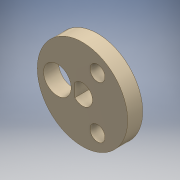
# Autodesk Inventor part: Carrier_top
Saved by Autodesk Inventor 2016 (Build 200138000, 138)
## iProperties
Created: 2015-12-09
Part Number: Carrier_top
Material: Generic
Document SubType Name: Modeling
Designer: lk8187
Density: 1 g/cm^3
Appearance: Smooth - Light Beige
Author: lk8187
Autodesk Inventor part; units mm, degrees
ref_plane "YZ Plane" through (0, 0, 0) normal (1, 0, 0) x (0, 1, 0)
ref_plane "XZ Plane" through (0, 0, 0) normal (0, 1, 0) x (-1, 0, 0)
ref_plane "XY Plane" through (0, 0, 0) normal (0, 0, 1) x (1, 0, 0)
sketch "Sketch1" plane through (0, 0, 0) normal (0, 1, 0) x (-1, 0, 0)
  circle A0 centre (0, 0) radius 9
  circle A1 centre (5, 0) radius 6 construction
  line L0 (0, 0) -> (-3, -5.1962) construction
  line L1 (0, 0) -> (-3, 5.1962) construction
  line L2 (0, 0) -> (-6.6506, 0) construction
  circle A2 centre (-3, 5.1962) radius 1.5
  circle A3 centre (-3, -5.1962) radius 1.5
  circle A4 centre (5, 0) radius 2.75
  arc A5 (1.5, 1.3229) -> (1.5, -1.3229) centre (0, 0) ccw
  line L3 (1.5, 1.3229) -> (1.5, -1.3229)
  dimension "d0" = 18
  dimension "d1" = 5
  dimension "d2" = 12
  dimension "d3" = 60
  dimension "d4" = 6
  dimension "d5" = 3
  dimension "d6" = 3
  dimension "d7" = 5.5
  dimension "d9" = 4
  dimension "d10" = 1.5
  constraints: 8 end point, 6 centre point, 5 coincident, 2 point on circle, 1 equal length, 1 horizontal, 1 horizontal alignment, 1 vertical, 1 vertical alignment
  measures "d0" diameter of A0
  measures "d1" distance of A1.centre point (0, 0)
  measures "d2" diameter of A1
  measures "d3" angle of L2 L0
  measures "d4" distance of L0.start L0.end
  measures "d5" diameter of A3
  measures "d6" diameter of A2
  measures "d7" diameter of A4
  measures "d9" diameter of A5
  measures "d10" distance from line of L3 point (0, 0)
extrude "Extrusion1" add sketch "Sketch1" against normal blind 3
body "Solid1"
